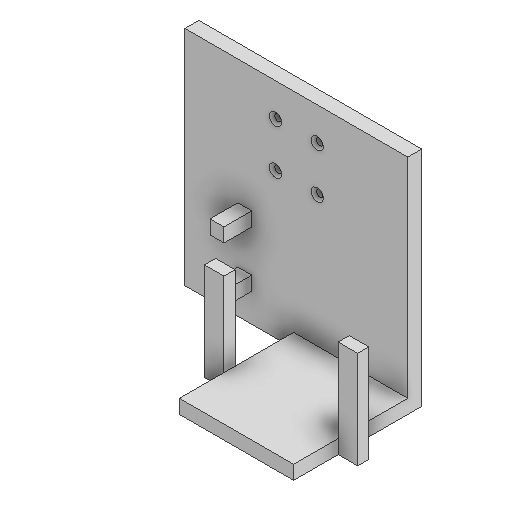
# Autodesk Inventor part: podstawa_rysika
Saved by Autodesk Inventor 2025.1 (Build 291241000, 241)
## iProperties
Created: 2025-04-09
Part Number: podstawa_rysika
Material: Ogólny
Document SubType Name: Modeling
Designer: Maciej
Density: 1 g/cm^3
Appearance: Domyślna
Author: Maciej
Autodesk Inventor part; units mm, degrees
ref_plane "YZ Plane" through (0, 0, 0) normal (1, 0, 0) x (0, 1, 0)
ref_plane "XZ Plane" through (0, 0, 0) normal (0, 1, 0) x (-1, 0, 0)
ref_plane "XY Plane" through (0, 0, 0) normal (0, 0, 1) x (1, 0, 0)
sketch "Szkic1" plane through (0, 0, 0) normal (0, 0, 1) x (1, 0, 0)
  line L0 (0, 0) -> (80, 0)
  line L1 (80, 0) -> (80, 80)
  line L2 (80, 80) -> (0, 80)
  line L3 (0, 80) -> (0, 0)
  dimension "d0" = 80
  dimension "d1" = 80
  constraints: 8 end point, 2 parallel, 1 horizontal, 1 perpendicular
  measures "d0" distance of L2.end L1.end
  measures "d1" distance of L1.end L0.end
extrude "Wyciągnięcie proste1" add sketch "Szkic1" along normal blind 5
sketch "Szkic2" plane through (0, 0, 5) normal (0, 0, 1) x (1, 0, 0)
  line L0 (80, 0) -> (80, 80) projected
  line L1 (80, 0) -> (39, 0)
  line L2 (39, 0) -> (39, 5)
  line L3 (39, 5) -> (80, 5)
  line L4 (80, 5) -> (80, 0)
  point P0 (0, 0)
  dimension "d6" = 41
  dimension "d7" = 5
  constraints: 8 end point, 2 parallel, 1 horizontal, 1 perpendicular
  measures "d6" distance of L2.end L3.end
  measures "d7" distance of L1.end L2.end
extrude "Wyciągnięcie proste2" add sketch "Szkic2" along normal blind 41
sketch "Szkic3" plane through (0, 0, 5) normal (0, 0, 1) x (1, 0, 0)
  line L0 (19, 35.2968) -> (24, 35.2968)
  line L1 (24, 35.2968) -> (24, 30.2968)
  line L2 (24, 30.2968) -> (19, 30.2968)
  line L3 (19, 30.2968) -> (19, 35.2968)
  line L4 (19, 15.2968) -> (24, 15.2968)
  line L5 (24, 15.2968) -> (24, 10.2968)
  line L6 (24, 10.2968) -> (19, 10.2968)
  line L7 (19, 10.2968) -> (19, 15.2968)
  line L8 (39, 5) -> (39, 0) projected
  point P0 (0, 0)
  point P1 (39, 2.5)
  point P2 (24, 12.7968)
  dimension "d10" = 5
  dimension "d11" = 5
  dimension "d12" = 5
  dimension "d13" = 15
  dimension "d14" = 15
  constraints: 16 end point, 4 parallel, 2 horizontal, 2 midpoint, 2 perpendicular, 2 point on line
  measures "d10" distance of L1.end L2.end
  measures "d11" distance of L0.end L1.end
  measures "d12" distance of L4.end L5.end
  measures "d13" distance of L4.end L1.end
  measures "d14" horizontal distance of point (39, 2.5) point (24, 12.797)
extrude "Wyciągnięcie proste3" add sketch "Szkic3" along normal blind 10
sketch "Szkic4" plane through (0, 0, 5) normal (0, 0, 1) x (1, 0, 0)
  line L0 (80, 80) -> (0, 80) projected
  line L1 (80, 5) -> (80, 80) projected
  point P0 (0, 0)
  point P1 (32.5, 68.05)
  point P2 (47.5, 68.05)
  point P3 (47.5, 52.05)
  point P4 (32.5, 52.05)
  dimension "d17" = 11.95
  dimension "d18" = 11.95
  dimension "d19" = 15
  dimension "d20" = 15
  dimension "d21" = 16
  dimension "d22" = 16
  dimension "d23" = 32.5
  dimension "d24" = 32.5
  measures "d17" distance from line of L0 point (32.5, 68.05)
  measures "d18" distance from line of L0 point (47.5, 68.05)
  measures "d19" distance of point (47.5, 68.05) point (32.5, 68.05)
  measures "d20" distance of point (47.5, 52.05) point (32.5, 52.05)
  measures "d21" distance of point (32.5, 68.05) point (32.5, 52.05)
  measures "d22" distance of point (47.5, 68.05) point (47.5, 52.05)
  measures "d23" distance from line of L1 point (47.5, 68.05)
  measures "d24" distance from line of L1 point (47.5, 52.05)
hole "Otwór1" at (32.5, 68.05, 5) at (47.5, 68.05, 5) at (47.5, 52.05, 5) at (32.5, 52.05, 5) direction (0, 0, -1) diameter 2.5 depth 5 tip angle 118 countersink diameter 4.4 countersink angle 90 clearance for "Śruba ze łbem płaskim obrobiona" size "M2" standard "ANSI Profil metryczny M"
sketch "Szkic5" plane through (39, 0, 5) normal (-1, 0, 0) x (0, 0, 1)
  line L0 (-5, 0) -> (41, 0) projected
  line L1 (21, 0) -> (25, 0)
  line L2 (25, 0) -> (25, 35)
  line L3 (25, 35) -> (21, 35)
  line L4 (21, 35) -> (21, 0)
  line L5 (0, 80) -> (0, 0) projected
  dimension "d32" = 4
  dimension "d33" = 35
  dimension "d34" = 21
  constraints: 8 end point, 2 parallel, 1 horizontal, 1 perpendicular, 1 point on line
  measures "d32" distance of L3.end L2.end
  measures "d33" distance of L2.end L1.end
  measures "d34" distance between parallel lines of L5 L4
extrude "Wyciągnięcie proste4" add sketch "Szkic5" along normal blind 7
sketch "Szkic6" plane through (80, 0, 0) normal (1, 0, 0) x (0, 0, -1)
  line L0 (-30, 5) -> (-30, 35) projected
  line L1 (-5, 0) -> (-26, 0) projected
  line L2 (-30, 35) -> (-26, 35)
  line L3 (-26, 35) -> (-26, 0)
  line L4 (-26, 0) -> (-30, 0)
  line L5 (-30, 0) -> (-30, 35)
  point P0 (0, 0)
  point P1 (-30, 5)
  constraints: 8 end point, 2 parallel, 1 horizontal, 1 perpendicular
extrude "Wyciągnięcie proste5" add sketch "Szkic6" along normal blind 7
equation "\"d18\" = d17"
equation "\"d22\" = d21"
equation "\"d24\" = d23"
